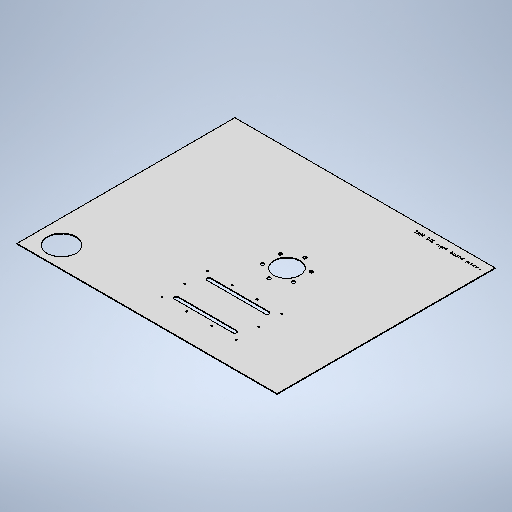
# Autodesk Inventor part: TRM 016 right board main++
Saved by Autodesk Inventor 2025 (Build 290162010, 162A)
## iProperties
Created: 2024-08-07
Part Number: TRM 016 right board main++
Material: AISI 304
Document SubType Name: Sheet Metal
Designer: pokla
Stock Number: ТРМ 015 левый борт основное
Density: 8.02768 g/cm^3
Flat Pattern Width: 67 cm
Flat Pattern Length: 80 cm
Flat Pattern Area: 5360 cm^2
Sheet Metal Rule: AISI304 2mm Die16
Sheet Metal Width: 670,000 mm
Sheet Metal Length: 800,000 mm
Sheet Metal Area: 536000,000 mm^2
Appearance: Default
Author: pokla
Autodesk Inventor part; units mm, degrees
ref_plane "YZ Plane" through (0, 0, 0) normal (1, 0, 0) x (0, 1, 0)
ref_plane "XZ Plane" through (0, 0, 0) normal (0, 1, 0) x (-1, 0, 0)
ref_plane "XY Plane" through (0, 0, 0) normal (0, 0, 1) x (1, 0, 0)
sketch "Sketch1" plane through (0, 0, 0) normal (0, 0, 1) x (1, 0, 0)
  line L0 (320, 0) -> (320, 670)
  line L1 (320, 670) -> (-480, 670)
  line L2 (-480, 670) -> (-480, 0)
  circle A0 centre (0, 350) radius 40
  line L3 (320, 0) -> (-480, 0)
  point P0 (0, 0)
  dimension "d14" = 80
  dimension "d15" = 320
  dimension "d17" = 320
  dimension "d26" = 800
  dimension "d27" = 670
  measures "d14" diameter of A0
  measures "d15" distance from line of A0.centre L1
  measures "d17" distance from line of L0 A0.centre
  measures "d26" distance between parallel lines of L2 L0
  measures "d27" distance between parallel lines of L3 L1
extrude "Plate1" add sketch "Sketch1" along normal blind 2
sketch "Sketch3" plane through (0, 0, 2) normal (0, 0, 1) x (1, 0, 0)
  circle A0 centre (0, 405) radius 5
  circle A1 centre (0, 350) radius 40 projected
  point P0 (0, 0)
  dimension "d19" = 10
  dimension "d20" = 55
  constraints: 1 centre point, 1 vertical alignment
  measures "d19" diameter of A0
  measures "d20" distance of A1.centre A0.centre
extrude "Cut1" cut sketch "Sketch3" against normal through all contours A0
pattern_circular "Circular Pattern1" count 6 over 360 about axis through (0, 350, 0) along (0, 0, 1) of "Cut1"
sketch "Sketch4" plane through (0, 0, 2) normal (0, 0, 1) x (1, 0, 0)
  line L0 (100, 650) -> (300, 650) construction
  line L1 (300, 650) -> (300, 630) construction
  line L2 (300, 630) -> (100, 630) construction
  line L3 (100, 630) -> (100, 650) construction
  line L4 (-480, 670) -> (320, 670) projected
  line L5 (320, 670) -> (320, 0) projected
  point P0 (0, 0)
  dimension "d28" = 200
  dimension "d29" = 20
  dimension "d30" = 20
  dimension "d31" = 20
  constraints: 2 other
  measures "d28" distance of L3.end L0.end
  measures "d29" distance of L0.end L1.end
  measures "d30" distance between parallel lines of L4 L0
  measures "d31" distance between parallel lines of L5 L1
mark "Mark2"
sketch "Sketch5" plane through (-480, 670, 2) normal (0, 0, 1) x (1, 0, 0)
  circle A0 centre (72.8, -605.5) radius 44.5
  line L0 (0, -670) -> (0, 0) projected
  line L1 (800, -670) -> (0, -670) projected
  dimension "d32" = 72.8
  dimension "d33" = 89
  dimension "d34" = 64.5
  constraints: 1 centre point
  measures "d32" distance from line of L0 A0.centre
  measures "d33" diameter of A0
  measures "d34" distance from line of L1 A0.centre
extrude "Extrusion1" cut sketch "Sketch5" against normal through all
sketch "Sketch6" plane through (-480, 670, 2) normal (0, 0, 1) x (1, 0, 0)
  circle A0 centre (480, -320) radius 40 projected
  line L0 (480, -320) -> (480, -670) construction
  line L1 (0, -670) -> (800, -670) projected
  line L2 (390, -470) -> (570, -470) construction
  line L3 (390, -476) -> (570, -476)
  line L4 (570, -464) -> (390, -464)
  arc A1 (390, -464) -> (390, -476) centre (390, -470) ccw
  arc A2 (570, -476) -> (570, -464) centre (570, -470) ccw
  line L5 (390, -570) -> (570, -570) construction
  line L6 (390, -576) -> (570, -576)
  line L7 (570, -564) -> (390, -564)
  arc A3 (390, -564) -> (390, -576) centre (390, -570) ccw
  arc A4 (570, -576) -> (570, -564) centre (570, -570) ccw
  line L8 (480, -470) -> (480, -570) construction
  line L9 (366, -450) -> (594, -450) construction
  line L10 (594, -450) -> (594, -590) construction
  line L11 (594, -590) -> (366, -590) construction
  line L12 (366, -590) -> (366, -450) construction
  line L13 (366, -450) -> (594, -590) construction
  circle A5 centre (366, -450) radius 2.5
  line L14 (442, -450) -> (442, -590) construction
  line L15 (518, -450) -> (518, -590) construction
  circle A6 centre (442, -450) radius 2.5
  circle A7 centre (518, -450) radius 2.5
  circle A8 centre (594, -450) radius 2.5
  circle A9 centre (594, -520) radius 2.5
  circle A10 centre (594, -590) radius 2.5
  circle A11 centre (518, -590) radius 2.5
  circle A12 centre (442, -590) radius 2.5
  circle A13 centre (366, -590) radius 2.5
  circle A14 centre (366, -520) radius 2.5
  point P0 (480, -520)
  dimension "d37" = 180
  dimension "d38" = 12
  dimension "d41" = 100
  dimension "d42" = 150
  dimension "d43" = 228
  dimension "d45" = 5
  dimension "d46" = 140
  dimension "d47" = 76
  dimension "d48" = 76
  constraints: 34 end point, 14 centre point, 10 equal radius, 8 coincident, 8 point on circle, 8 tangent, 6 midpoint, 5 parallel, 5 perpendicular, 5 point on line, 2 vertical alignment, 1 horizontal, 1 vertical
  measures "d37" distance of L2.start L2.end
  measures "d38" diameter of A2
  measures "d41" distance of L8.start L8.end
  measures "d42" distance of point (480, -520) L0.end
  measures "d43" distance of L10.end L11.end
  measures "d45" diameter of A5
  measures "d46" distance of L11.end A5.centre
  measures "d47" distance between parallel lines of L12 L14
  measures "d48" distance of L10.end L15.end
extrude "Extrusion2" cut sketch "Sketch6" against normal through all contours A1 L4 A2 L3 | A3 L7 A4 L6 | A5 | A6 | A7 | A8 | A9 | A10 | A11 | A12 | A13 | A14
equation "\"d2\" = Thickness"
equation "\"BendReliefWidth\" = Thickness"
equation "\"BendReliefDepth\" = 0.5 * Thickness"
equation "\"CornerReliefSize\" = 4 * Thickness"
equation "\"MinimumRemnant\" = 2 * Thickness"
equation "\"TransitionRadius\" = BendRadius"
equation "\"JacobiRadiusSize\" = BendRadius"
equation "\"GapSize\" = Thickness"
equation "\"Thickness\" = 2"
equation "\"BendRadius\" = 2.75"
body "Solid1"
